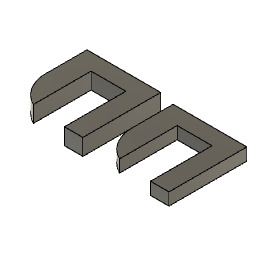
18650 battery cap (Autodesk Fusion 360 design; units mm, degrees)
Autodesk Fusion 360 part; units mm, degrees
sketch "Sketch1" plane through (0, 0, 0) normal (0, 0, 1) x (1, 0, 0)
  line L0 (9, 0) -> (18, 0)
  line L1 (18, 0) -> (18, 19)
  line L2 (18, 19) -> (0, 19)
  line L3 (0, 19) -> (0, 9)
  arc A0 (0, 9) -> (9, 0) centre (9, 9) ccw
  line L4 (5, 0) -> (5, 15)
  line L5 (5, 15) -> (13.5, 15)
  line L6 (13.5, 15) -> (13.5, 0)
  constraint horizontal L0
  constraint vertical L1
  constraint horizontal L2
  constraint vertical L3
  constraint coincident origin L0
  constraint coincident origin L3
  constraint tangent L0 A0
  constraint tangent L3 A0
  constraint vertical L4
  constraint horizontal L5
  constraint vertical L6
  constraint coincident L0 L6.end
extrude "Extrude1" add sketch "Sketch1" along normal blind 4 contours L0 L1 L2 L3 A0 L4 L5 L6 makes body 1
copy_body "CopyPasteBodies1" bodies 1 makes body 2
move_body "Move1" bodies 2 to x (1, 0, 0) y (0, 1, 0) z (0, 0, 1) at (21, 0, 0)
move_face "OffsetFaces1" offset -1 1 faces at (37.5, 11.3333, 4) on bodies 2
